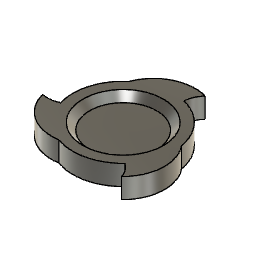
blade_sketch (Autodesk Fusion 360 design; units mm, degrees)
Autodesk Fusion 360 part; units mm, degrees
note: some values were not read from the file. Set by a fixed rule: which sketch regions a step uses.
sketch "Sketch1" plane through (0, 0, 0) normal (0, 0, 1) x (1, 0, 0)
  circle A0 centre (0, 0) radius 15
  dimension "d1" = 30
  constraint coincident A0.centre origin
  measures "d1" diameter of A0
extrude "Extrude1" add sketch "Sketch1" along normal blind 6
sketch "Sketch2" plane through (0, 0, 6) normal (0, 0, 1) x (-1, 0, 0)
  circle A0 centre (0, 0) radius 15
  circle A1 centre (-2, -7) radius 12.5
  circle A2 centre (-11, -14) radius 7.5
  dimension "d4" = 25
  dimension "d5" = 15
  dimension "d6" = 7
  dimension "d7" = 2
  dimension "d8" = 14
  dimension "d9" = 11
  measures "d4" diameter of A1
  measures "d5" diameter of A2
  measures "d6" vertical distance of A0.centre A1.centre
  measures "d7" horizontal distance of A0.centre A1.centre
  measures "d8" vertical distance of A0.centre A2.centre
  measures "d9" horizontal distance of A0.centre A2.centre
extrude "Extrude2" add sketch "Sketch2" against normal blind 6 contours A0 A1 A2 picked at (-2.4117, -16.9728)
pattern_circular "C-Pattern1" count 3 over 360 about axis through (0, 0, 6) along (0, 0, 1) of "Extrude2"
sketch "Sketch3" plane through (0, 0, 6) normal (0, 0, 1) x (-1, 0, 0)
  arc A0 (9.6768, -11.4612) -> (14.3884, 4.2397) centre (0, 0) ccw
  arc A1 (19.1866, 4.8092) -> (14.3884, 4.2397) centre (17.6244, -2.5263) ccw
  arc A2 (19.1866, 4.8092) -> (5.0873, 14.111) centre (7.0622, 1.7679) ccw
  arc A3 (5.0873, 14.111) -> (-10.8659, 10.3408) centre (0, 0) ccw
  arc A4 (-13.7582, 14.2114) -> (-10.8659, 10.3408) centre (-6.6244, 16.5263) ccw
  arc A5 (-13.7582, 14.2114) -> (-14.7641, -2.6497) centre (-5.0622, 5.2321) ccw
  arc A6 (-14.7641, -2.6497) -> (-3.5225, -14.5805) centre (0, 0) ccw
  arc A7 (-5.4284, -19.0207) -> (-3.5225, -14.5805) centre (-11, -14) ccw
  arc A8 (-5.4284, -19.0207) -> (9.6768, -11.4612) centre (-2, -7) ccw
  circle A9 centre (0, 0) radius 12
  dimension "d14" = 24
  constraint coincident A0.centre A3.centre
  measures "d14" diameter of A9
extrude "Extrude3" cut sketch "Sketch3" against normal blind 2 draft -45 contours A9
